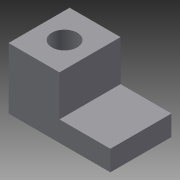
# Autodesk Inventor part: SamplePart
Saved by Autodesk Inventor 2014 Beta1 (Build 180079000, 79) ContinuousBuild 0
## iProperties
Created: 2012-10-03
Part Number: SamplePart
Material: Generic
Document SubType Name: Modeling
Designer: ekinsb
Density: 1 g/cm^3
Appearance: Default
Author: ekinsb
Autodesk Inventor part; units mm, degrees
ref_plane "YZ Plane" through (0, 0, 0) normal (1, 0, 0) x (0, 1, 0)
ref_plane "XZ Plane" through (0, 0, 0) normal (0, 1, 0) x (-1, 0, 0)
ref_plane "XY Plane" through (0, 0, 0) normal (0, 0, 1) x (1, 0, 0)
sketch "Sketch1" plane through (0, 0, 0) normal (0, 0, 1) x (1, 0, 0)
  line L0 (0, 0) -> (127, 0)
  line L1 (127, 0) -> (127, 25.3956)
  line L2 (127, 25.3956) -> (63.5, 25.3956)
  line L3 (63.5, 25.3956) -> (63.5, 76.2)
  line L4 (63.5, 76.2) -> (0, 76.2)
  line L5 (0, 76.2) -> (0, 0)
  dimension "d0" = 127
  dimension "d16" = 63.5
  dimension "d17" = 25.3956
  dimension "d18" = 76.2
  constraints: 12 end point, 4 parallel, 1 horizontal, 1 perpendicular
  measures "d0" distance of L0.start L0.end
  measures "d16" distance of L3.end L4.end
  measures "d17" distance of L0.end L1.end
  measures "d18" distance of L4.end L0.start
extrude "Extrusion1" add sketch "Sketch1" along normal blind 76.2
sketch "Sketch2" plane through (0, 76.2, 0) normal (0, 1, 0) x (1, 0, 0)
  circle A0 centre (31.75, -38.1) radius 15.875
  dimension "d3" = 31.75
  constraints: 1 centre point
  measures "d3" diameter of A0
extrude "Extrusion2" cut sketch "Sketch2" against normal through all
body "Solid1"
